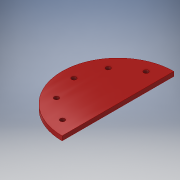
# Autodesk Inventor part: SupportPlateForWaterHalf
Saved by Autodesk Inventor 2019 (Build 230136000, 136)
## iProperties
Created: 2017-11-20
Part Number: SupportPlateForWaterHalf
Material: PET Plastic
Document SubType Name: Modeling
Designer: steele
Density: 1.541 g/cm^3
Appearance: Red
Author: steele
Autodesk Inventor part; units mm, degrees
ref_plane "YZ Plane" through (0, 0, 0) normal (1, 0, 0) x (0, 1, 0)
ref_plane "XZ Plane" through (0, 0, 0) normal (0, 1, 0) x (-1, 0, 0)
ref_plane "XY Plane" through (0, 0, 0) normal (0, 0, 1) x (1, 0, 0)
sketch "Sketch1" plane through (0, 0, 0) normal (0, 1, 0) x (-1, 0, 0)
  circle A0 centre (0, 0) radius 80.645
  dimension "d4" = 161.29
  constraints: 1 centre point, 1 coincident
  measures "d4" diameter of A0
extrude "Extrusion1" add sketch "Sketch1" against normal blind 6.35
sketch "Sketch2" plane through (0, 0, 0) normal (0, 1, 0) x (1, 0, 0)
  arc A0 (0, -80.645) -> (0, 80.645) centre (0, 0) ccw
  circle A1 centre (0, 0) radius 80.645 projected
  line L0 (0, 80.645) -> (0, -80.645)
  constraints: 4 point on circle, 2 end point, 1 centre point, 1 coincident, 1 vertical
extrude "Extrusion2" cut sketch "Sketch2" against normal through all contours L0 A0
sketch "Sketch5" plane through (0, 0, 0) normal (0, 1, 0) x (1, 0, 0)
  circle A0 centre (0, 0) radius 63.5 construction
  circle A1 centre (-63.5, 0) radius 3.3782
  circle A2 centre (-51.3726, -37.3244) radius 3.3782
  circle A3 centre (-19.6226, -60.3921) radius 3.3782
  circle A4 centre (19.6226, -60.3921) radius 3.3782
  circle A5 centre (51.3726, -37.3244) radius 3.3782
  circle A6 centre (63.5, 0) radius 3.3782
  circle A7 centre (51.3726, 37.3244) radius 3.3782
  circle A8 centre (19.6226, 60.3921) radius 3.3782
  circle A9 centre (-19.6226, 60.3921) radius 3.3782
  circle A10 centre (-51.3726, 37.3244) radius 3.3782
  dimension "d17" = 127
  dimension "d18" = 6.7564
  dimension "d21" = 360
  constraints: 10 centre point, 1 coincident, 1 horizontal alignment, 23 other
  measures "d18" diameter of A1
extrude "Extrusion3" cut sketch "Sketch5" against normal through all contours A1 | A2 | A3 | A9 | A10
body "Solid1"
